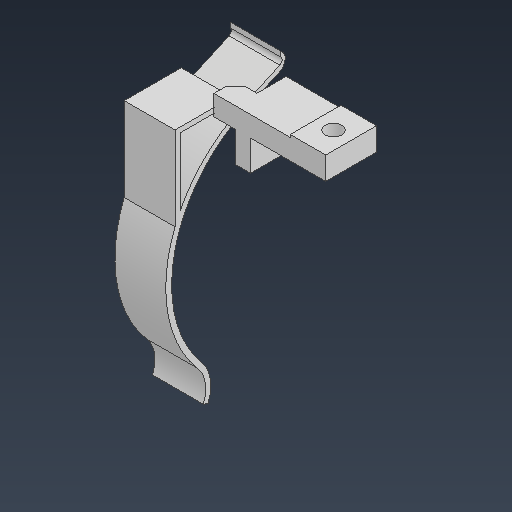
# Autodesk Inventor part: spool_blocker
Saved by Autodesk Inventor 2025.2 (Build 292293000, 293)
## iProperties
Created: 2025-02-27
Part Number: spool_blocker
Material: Generic
Document SubType Name: Modeling
Designer: email
Density: 1 g/cm^3
Appearance: Default
Author: email
Autodesk Inventor part; units mm, degrees
ref_plane "YZ Plane" through (0, 0, 0) normal (1, 0, 0) x (0, 1, 0)
ref_plane "XZ Plane" through (0, 0, 0) normal (0, 1, 0) x (-1, 0, 0)
sketch "Sketch2" plane through (0, 0, 0) normal (0, 1, 0) x (-1, 0, 0)
  line L0 (0, 0) -> (-7, 0)
  line L1 (-7, 0) -> (-7, -10)
  line L2 (-7, -10) -> (0, -10)
  line L3 (0, -10) -> (0, 0)
  circle A0 centre (-3.5, -5) radius 1.65
  line L4 (0, 0) -> (15, 0)
  line L5 (15, 0) -> (15, -15.9854)
  line L6 (15, -15.9854) -> (0, -15.9854)
  line L7 (0, -15.9854) -> (0, 0)
  line L8 (7.8, 0) -> (10.8, 0)
  line L9 (10.8, 0) -> (10.8, -15.9854)
  line L10 (10.8, -15.9854) -> (7.8, -15.9854)
  line L11 (7.8, -15.9854) -> (7.8, 0)
  line L12 (15, -15.9854) -> (10.8, -15.9854)
  line L13 (10.8, -15.9854) -> (10.8, -4.2527)
  line L14 (10.8, -4.2527) -> (15, -4.2527)
  line L15 (15, -4.2527) -> (15, -15.9854)
  line L16 (0, -10) -> (10.8, -10)
  point P0 (0, -5)
  point P1 (-3.5, -10)
  point P2 (10.8, 0)
  point P3 (15, -4.2527)
  point P4 (7.8, -10)
  dimension "d2" = 7
  dimension "d3" = 10
  dimension "d4" = 3.3
  dimension "d12" = 22
  dimension "d21" = 11.3
  dimension "d22" = 3
  constraints: 34 end point, 8 parallel, 5 perpendicular, 4 horizontal, 4 point on line, 2 midpoint, 1 centre point, 1 horizontal alignment, 1 vertical alignment
  measures "d2" distance of L1.end L2.end
  measures "d3" distance of L0.end L1.end
  measures "d4" diameter of A0
  measures "d12" distance between parallel lines of L5 L1
  measures "d21" distance from line of A0.centre L11
  measures "d22" distance between parallel lines of L9 L11
extrude "Extrusion1" add sketch "Sketch2" along normal blind 4.5 contours L3 L2 L1 L0
extrude "Extrusion2" add sketch "Sketch2" along normal blind 4 contours L4 L11 L16 L3 | L4 L9 L16 L11 | L4 L5 L14 L9
ref_plane "Work Plane1" through (0, 0, 0) normal (0, -0.9396926, -0.3420201) x (-1, 0, 0)
sketch "Sketch4" plane through (-15, 0, -15.9854) normal (-1, 0, 0) x (0, 0, 1)
  line L0 (-0.8784, 3) -> (12.8006, -3.1551)
  line L1 (12.8006, -3.1551) -> (13.2109, -2.2432)
  line L2 (13.2109, -2.2432) -> (-0.4681, 3.9119)
  line L3 (-0.8784, 3) -> (-0.4681, 3.9119)
  arc A0 (18.4229, -40.6351) -> (9.5813, -1.7065) centre (-0.6772, -24.5048) ccw
  line L4 (18.4229, -40.6351) -> (19.1869, -41.2803)
  line L5 (9.5813, -1.7065) -> (10.2986, -0.9327)
  arc A1 (19.1869, -41.2803) -> (10.2986, -0.9327) centre (-0.2668, -24.413) ccw
  arc A2 (18.4229, -40.6351) -> (17.1504, -48.2979) centre (24.2261, -45.5359) ccw
  arc A3 (19.1869, -41.2803) -> (18.0819, -47.9342) centre (24.064, -45.509) ccw
  line L6 (17.1504, -48.2979) -> (18.0819, -47.9342)
  line L7 (22.6596, -12.694) -> (22.6596, 0.6055)
  line L8 (22.6596, 0.6055) -> (12.4332, 0.6055)
  line L9 (12.4332, 0.6055) -> (12.4332, 1.6055)
  line L10 (12.4332, 1.6055) -> (23.6596, 1.6055)
  line L11 (23.6596, 1.6055) -> (23.6596, -14.9008)
  line L12 (5.9854, 0) -> (11.7327, 0) projected
  arc A4 (2.815, 4.6033) -> (3.1019, 1.209) centre (3.9014, 2.9858) ccw
  line L13 (2.815, 4.6033) -> (2.815, 3.6033)
  arc A5 (2.815, 3.6033) -> (3.0226, 2.3412) centre (3.3375, 3.0411) ccw
  point P0 (15.9854, 0)
  point P1 (13.4215, -1.7995)
  point P2 (1.9601, 2.8193)
  point P3 (2.654, 2.6401)
  dimension "d14" = 1
  dimension "d20" = 15
  dimension "d26" = 25
  dimension "d27" = 1
  dimension "d29" = 1
  dimension "d30" = 1
  dimension "d31" = 1
  dimension "d35" = 3
  dimension "d37" = 1
  dimension "d38" = 1
  constraints: 26 end point, 14 point on circle, 6 centre point, 6 perpendicular, 6 tangent, 4 point on line, 2 line through centre, 2 vertical
  measures "d14" distance between parallel lines of L0 L2
  measures "d20" distance of L1.end L2.end
  measures "d26" radius of A0
  measures "d27" distance of L4.start L4.end
  measures "d29" distance of L6.start L6.end
  measures "d30" distance between parallel lines of L11 L7
  measures "d31" distance between parallel lines of L10 L8
  measures "d35" distance from line of L12 L0.start
  measures "d37" distance of L0.start L2.end
  measures "d38" distance of L13.start L13.end
extrude "Extrusion4" add sketch "Sketch4" along normal blind 10 contours A4 L2 L5 L0 | L5 A1 L1 L0 | L0 L1 A1 L4 A0 | A4 L13 A5 L2 | L4 A3 L6 A2 | L7 L8 L9 L10 L11 A1
extrude "Extrusion5" add sketch "Sketch2" against normal blind 6 contours L4 L9 L16 L11
chamfer "Chamfer1" distance 2 angle 45 1 edges at (-15, 2, -4.2527)
body "Solid1"
